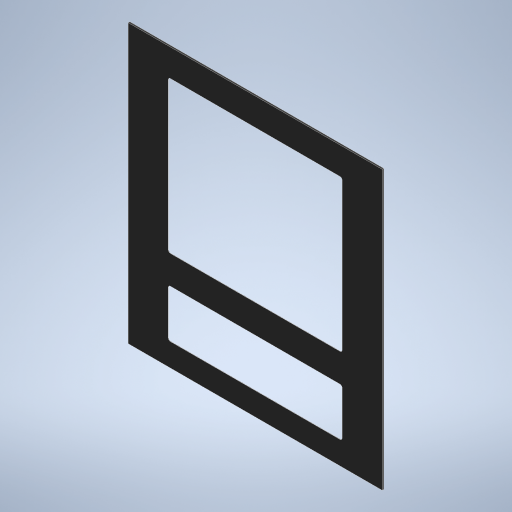
# Autodesk Inventor part: Door Panel
Saved by Autodesk Inventor 2024 (Build 280153000, 153)
## iProperties
Created: 2024-09-03
Part Number: Door Panel
Material: PET Plastic
Document SubType Name: Modeling
Designer: Ishaan
Density: 1.541 g/cm^3
Appearance: Polycarbonate - Clear
Author: Ishaan
Autodesk Inventor part; units mm, degrees
ref_plane "YZ Plane" through (0, 0, 0) normal (1, 0, 0) x (0, 1, 0)
ref_plane "XZ Plane" through (0, 0, 0) normal (0, 1, 0) x (-1, 0, 0)
ref_plane "XY Plane" through (0, 0, 0) normal (0, 0, 1) x (1, 0, 0)
sketch "Sketch1" plane through (0, 0, 0) normal (0, 0, 1) x (1, 0, 0)
  line L0 (233, -255) -> (-233, -255)
  line L1 (-233, -255) -> (-233, 255)
  line L2 (-233, 255) -> (233, 255)
  line L3 (233, 255) -> (233, -255)
  line L4 (233, -255) -> (-233, 255) construction
  line L5 (-233, -255) -> (233, 255) construction
  point P0 (0, 0)
  dimension "d0" = 466
  dimension "d1" = 510
  constraints: 12 end point, 2 midpoint, 2 parallel, 1 horizontal, 1 perpendicular
  measures "d0" distance of L1.end L2.end
  measures "d1" distance of L0.end L1.end
extrude "Extrusion1" add sketch "Sketch1" against normal blind 3
sketch "Sketch2" plane through (0, 0, 0) normal (0, 0, 1) x (1, 0, 0)
  line L0 (159.5, -73) -> (-159.5, -73)
  line L1 (-159.5, -73) -> (-159.5, 205)
  line L2 (-159.5, 205) -> (159.5, 205)
  line L3 (159.5, 205) -> (159.5, -73)
  line L4 (159.5, -73) -> (-159.5, 205) construction
  line L5 (-159.5, -73) -> (159.5, 205) construction
  line L6 (-233, 255) -> (-233, -255) projected
  line L7 (233, -255) -> (233, 255) projected
  line L8 (233, 255) -> (-233, 255) projected
  line L9 (159.5, -213) -> (-159.5, -213)
  line L10 (-159.5, -213) -> (-159.5, -125)
  line L11 (-159.5, -125) -> (159.5, -125)
  line L12 (159.5, -125) -> (159.5, -213)
  line L13 (159.5, -213) -> (-159.5, -125) construction
  line L14 (-159.5, -213) -> (159.5, -125) construction
  point P0 (0, 0)
  point P1 (0, 66)
  point P2 (0, -169)
  dimension "d4" = 73.5
  dimension "d6" = 50
  dimension "d7" = 278
  dimension "d8" = 52
  dimension "d9" = 88
  constraints: 24 end point, 4 midpoint, 4 parallel, 2 collinear, 2 horizontal, 2 perpendicular, 1 vertical alignment
  measures "d4" distance between parallel lines of L1 L6
  measures "d6" distance between parallel lines of L8 L2
  measures "d7" distance between parallel lines of L0 L2
  measures "d8" distance between parallel lines of L0 L11
  measures "d9" distance between parallel lines of L11 L9
extrude "Extrusion2" cut sketch "Sketch2" against normal through all
fillet "Fillet1" radius 4 8 edges at (-159.5, 205, -1.5) (159.5, 205, -1.5) (159.5, -73, -1.5) (-159.5, -73, -1.5) (-159.5, -125, -1.5) (159.5, -125, -1.5) (159.5, -213, -1.5) (-159.5, -213, -1.5)
sketch "Sketch3" plane through (0, 0, -3) normal (0, 0, -1) x (-1, 0, 0)
  line L0 (159.5, -129) -> (159.5, -209) projected
  arc A0 (155.5, -213) -> (159.5, -209) centre (155.5, -209) ccw projected
  line L1 (155.5, -213) -> (-155.5, -213) projected
  arc A1 (-159.5, -209) -> (-155.5, -213) centre (-155.5, -209) ccw projected
  line L2 (-159.5, -209) -> (-159.5, -129) projected
  arc A2 (-155.5, -125) -> (-159.5, -129) centre (-155.5, -129) ccw projected
  line L3 (-155.5, -125) -> (155.5, -125) projected
  arc A3 (159.5, -129) -> (155.5, -125) centre (155.5, -129) ccw projected
  line L4 (159.5, 201) -> (159.5, -69) projected
  arc A4 (155.5, -73) -> (159.5, -69) centre (155.5, -69) ccw projected
  line L5 (155.5, -73) -> (-155.5, -73) projected
  arc A5 (-159.5, -69) -> (-155.5, -73) centre (-155.5, -69) ccw projected
  line L6 (-159.5, -69) -> (-159.5, 201) projected
  arc A6 (-155.5, 205) -> (-159.5, 201) centre (-155.5, 201) ccw projected
  line L7 (-155.5, 205) -> (155.5, 205) projected
  arc A7 (159.5, 201) -> (155.5, 205) centre (155.5, 201) ccw projected
  line L8 (233, 255) -> (-233, 255) projected
  line L9 (-233, 255) -> (-233, -255) projected
  line L10 (-233, -255) -> (233, -255) projected
  line L11 (233, -255) -> (233, 255) projected
  line L12 (-174.5, 201) -> (-174.5, -69)
  arc A8 (-174.5, -69) -> (-155.5, -88) centre (-155.5, -69) ccw
  line L13 (-155.5, -88) -> (155.5, -88)
  arc A9 (155.5, -88) -> (174.5, -69) centre (155.5, -69) ccw
  line L14 (174.5, -69) -> (174.5, 201)
  arc A10 (174.5, 201) -> (155.5, 220) centre (155.5, 201) ccw
  line L15 (155.5, 220) -> (-155.5, 220)
  arc A11 (-155.5, 220) -> (-174.5, 201) centre (-155.5, 201) ccw
  line L16 (155.5, -110) -> (-155.5, -110)
  arc A12 (-155.5, -110) -> (-174.5, -129) centre (-155.5, -129) ccw
  line L17 (-174.5, -129) -> (-174.5, -209)
  arc A13 (-174.5, -209) -> (-155.5, -228) centre (-155.5, -209) ccw
  line L18 (-155.5, -228) -> (155.5, -228)
  arc A14 (155.5, -228) -> (174.5, -209) centre (155.5, -209) ccw
  line L19 (174.5, -209) -> (174.5, -129)
  arc A15 (174.5, -129) -> (155.5, -110) centre (155.5, -129) ccw
  point P0 (0, 0)
  dimension "d13" = 15
  dimension "d14" = 15
  constraints: 16 end point, 16 point on circle, 8 centre point, 14 other
  measures "d13" radial gap between concentric circles of A6 A11
  measures "d14" distance between parallel lines of L3 L16
extrude "Extrusion3" cut sketch "Sketch3" against normal blind 2.3813 contours A11 L15 A10 L14 A9 L13 A8 L12 | A15 L19 A14 L18 A13 L17 A12 L16
body "Solid1"
